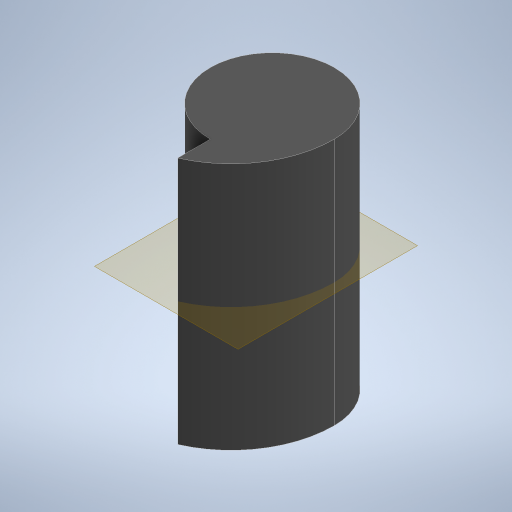
# Autodesk Inventor part: Drum
Saved by Autodesk Inventor 2024 (Build 280153000, 153)
## iProperties
Created: 2023-10-18
Part Number: Drum
Material: Generic
Document SubType Name: Modeling
Designer: CJ110
Density: 1 g/cm^3
Appearance: Default
Author: CJ110
Autodesk Inventor part; units mm, degrees
ref_plane "YZ Plane" through (0, 0, 0) normal (1, 0, 0) x (0, 1, 0)
ref_plane "XZ Plane" through (0, 0, 0) normal (0, 1, 0) x (-1, 0, 0)
ref_plane "XY Plane" through (0, 0, 0) normal (0, 0, 1) x (1, 0, 0)
sketch "Sketch1" plane through (0, 0, 0) normal (0, 1, 0) x (-1, 0, 0)
  circle A0 centre (0, 0) radius 24.13
  line L0 (0, 24.13) -> (0, 36.83)
  line L1 (0, 0) -> (0, 24.13) construction
  arc A1 (0, 36.83) -> (-24.13, 0) centre (16.0421, 0) ccw
  line L2 (0, 0) -> (-24.13, 0) construction
  dimension "d0" = 48.26
  dimension "d1" = 12.7
  constraints: 6 end point, 5 point on circle, 2 centre point, 2 vertical, 1 coincident, 1 collinear, 1 horizontal, 1 tangent
  measures "d0" diameter of A0
  measures "d1" distance of L0.start L0.end
extrude "Extrusion1" add sketch "Sketch1" along normal blind 96.52
ref_plane "Work Plane1" through (0, 48.26, 0) normal (0, 1, 0) x (1, 0, 0)
body "Solid1"
